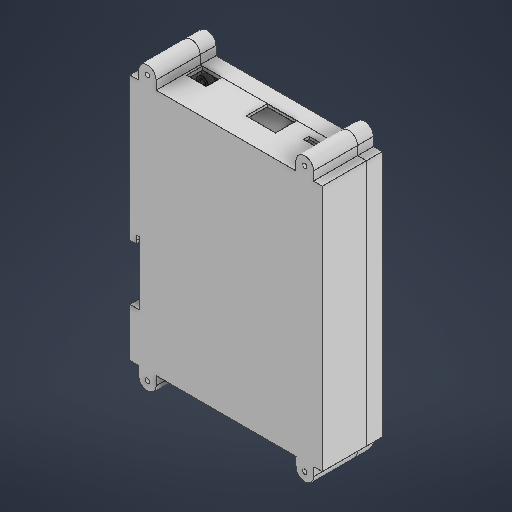
# Autodesk Inventor part: module_base
Saved by Autodesk Inventor 2025 (Build 290162000, 162)
## iProperties
Created: 2024-08-31
Part Number: module_base
Material: Generic
Document SubType Name: Modeling
Designer: Dawid
Density: 1 g/cm^3
Appearance: Default
Author: Dawid
Autodesk Inventor part; units mm, degrees
ref_plane "YZ Plane" through (0, 0, 0) normal (1, 0, 0) x (0, 1, 0)
ref_plane "XZ Plane" through (0, 0, 0) normal (0, 1, 0) x (-1, 0, 0)
ref_plane "XY Plane" through (0, 0, 0) normal (0, 0, 1) x (1, 0, 0)
sketch "Sketch1" plane through (0, 0, 0) normal (0, 0, 1) x (1, 0, 0)
  line L0 (0, 0) -> (70, 0) construction
  line L1 (70, 0) -> (70, 133.34) construction
  line L2 (70, 133.34) -> (0, 133.34) construction
  line L3 (0, 133.34) -> (0, 0) construction
  line L4 (-0.5, 133.84) -> (70.5, 133.84)
  line L5 (70.5, 133.84) -> (70.5, -3)
  line L6 (70.5, -3) -> (-26.344, -3)
  line L7 (-26.344, -3) -> (-26.344, 133.34)
  line L8 (-17.884, 58.58) -> (-12.804, 58.58) construction
  line L9 (-12.804, 58.58) -> (-12.804, 22.58) construction
  line L10 (-12.804, 22.58) -> (-17.884, 22.58) construction
  line L11 (-17.884, 22.58) -> (-17.884, 58.58) construction
  line L12 (-35.844, 135.34) -> (73.5, 135.34)
  line L13 (73.5, 135.34) -> (73.5, -5)
  line L14 (73.5, -5) -> (-35.844, -5)
  line L15 (-31.844, 58.58) -> (-30.344, 58.58)
  line L16 (-30.344, 58.58) -> (-30.344, 22.58)
  line L17 (-30.344, 22.58) -> (-35.844, 22.58)
  line L18 (-35.844, 54.08) -> (-35.844, 135.34)
  line L19 (-35.844, 54.08) -> (-32.144, 54.08)
  line L20 (-31.844, 56.08) -> (-31.844, 58.58)
  line L21 (-35.844, -5) -> (-35.844, 22.58)
  line L22 (-32.144, 54.08) -> (-31.844, 56.08)
  line L23 (-27, 133.34) -> (-1, 133.34) construction
  line L24 (-1, 133.34) -> (-1, 81.44) construction
  line L25 (-1, 81.44) -> (-27, 81.44) construction
  line L26 (-27, 81.44) -> (-27, 133.34) construction
  line L27 (-26.094, 68.63) -> (-4.594, 68.63) construction
  line L28 (-4.594, 68.63) -> (-4.594, 12.53) construction
  line L29 (-4.594, 12.53) -> (-26.094, 12.53) construction
  line L30 (-26.094, 12.53) -> (-26.094, 68.63) construction
  circle A0 centre (-21.62, 124.84) radius 3.5
  circle A1 centre (-6.38, 124.84) radius 3.5
  circle A2 centre (-21.62, 86.74) radius 3.5
  circle A3 centre (-6.38, 86.74) radius 3.5
  circle A4 centre (-21.694, 64.71) radius 3.5
  circle A5 centre (-8.994, 64.71) radius 3.5
  circle A6 centre (-21.694, 16.45) radius 3.5
  circle A7 centre (-8.994, 16.45) radius 3.5
  line L31 (-21.694, 64.71) -> (-8.994, 16.45) construction
  line L32 (-21.62, 124.84) -> (-6.38, 86.74) construction
  circle A8 centre (12.14, 104.13) radius 3.5
  circle A9 centre (57.86, 104.13) radius 3.5
  circle A10 centre (10.87, 29.26) radius 3.5
  circle A11 centre (59.13, 27.96) radius 3.5
  circle A12 centre (26.11, 80.06) radius 3.5
  line L33 (12.14, 104.13) -> (57.86, 104.13) construction
  line L34 (10.87, 29.26) -> (59.13, 29.26) construction
  line L35 (59.13, 29.26) -> (59.13, 27.96) construction
  line L36 (-26.344, 133.34) -> (-0.5, 133.34)
  line L37 (-0.5, 133.34) -> (-0.5, 133.84)
  line L38 (-12.604, 58.78) -> (-18.084, 58.78)
  line L39 (-18.084, 58.78) -> (-18.084, 22.38)
  line L40 (-18.084, 22.38) -> (-12.604, 22.38)
  line L41 (-12.604, 22.38) -> (-12.604, 58.78)
  point P0 (-15.344, 58.58)
  point P1 (-12.804, 40.58)
  point P2 (-15.344, 22.58)
  point P3 (-33.994, 54.08)
  point P4 (-30.344, 40.58)
  point P5 (-15.344, 40.58)
  point P6 (-4.594, 40.58)
  point P7 (-15.344, 12.53)
  point P8 (-14, 105.79)
  point P9 (-14, 81.44)
  point P10 (35, 104.13)
  point P11 (35, 133.34)
  point P12 (35, 29.26)
  dimension "d9" = 70
  dimension "d75" = 0.5
  dimension "d76" = 0.5
  dimension "d77" = 3
  dimension "d83" = 36
  dimension "d84" = 5.08
  dimension "d87" = 3
  dimension "d88" = 1.5
  dimension "d89" = 2
  dimension "d117" = 36
  dimension "d118" = 1.5
  dimension "d121" = 0.3
  dimension "d122" = 2
  dimension "d123" = 4.5
  dimension "d124" = 4
  dimension "d125" = 15
  dimension "d126" = 4
  dimension "d147" = 48.26
  dimension "d148" = 12.7
  dimension "d149" = 56.1
  dimension "d150" = 7
  dimension "d151" = 21.5
  dimension "d152" = 7
  dimension "d153" = 51.9
  dimension "d154" = 26
  dimension "d155" = 15.24
  dimension "d156" = 38.1
  dimension "d158" = 5
  dimension "d159" = 1
  dimension "d160" = 0.5
  dimension "d163" = 7
  dimension "d164" = 45.72
  dimension "d165" = 48.26
  dimension "d166" = 1.3
  dimension "d167" = 24.07
  dimension "d168" = 13.97
  dimension "d169" = 29.21
  dimension "d170" = 76.17
  dimension "d171" = 133.34
  dimension "d182" = 96.844
  dimension "d183" = 45.58
  dimension "d184" = 2
  dimension "d185" = 0.5
  dimension "d215" = 0.2
  constraints: 84 end point, 16 parallel, 13 centre point, 13 midpoint, 11 horizontal, 10 equal radius, 9 perpendicular, 9 vertical alignment, 7 horizontal alignment, 1 collinear, 1 vertical, 3 other
  measures "d9" distance of L1.end L2.end
  measures "d75" distance between parallel lines of L5 L1
  measures "d76" distance between parallel lines of L4 L2
  measures "d77" distance between parallel lines of L6 L0
  measures "d83" distance of L10.end L8.start
  measures "d84" distance of L8.start L8.end
  measures "d87" distance between parallel lines of L13 L5
  measures "d88" distance between parallel lines of L12 L4
  measures "d89" distance between parallel lines of L14 L6
  measures "d117" distance of L15.end L16.end
  measures "d118" distance of L15.start L15.end
  measures "d121" distance from line of L20 L19.end
  measures "d122" vertical distance of L19.end L20.start
  measures "d123" distance from line of point (-33.994, 54.08) L15
  measures "d124" distance between parallel lines of L18 L20
  measures "d125" distance from line of point (-15.344, 58.58) L16
  measures "d126" distance between parallel lines of L7 L16
  measures "d147" distance of L31.end A5.centre
  measures "d148" distance of L31.start A5.centre
  measures "d149" distance of L27.end L28.end
  measures "d150" diameter of A4
  measures "d151" distance of L27.start L27.end
  measures "d152" diameter of A0
  measures "d153" distance of L23.end L24.end
  measures "d154" distance of L24.end L25.end
  measures "d155" distance of L32.end A2.centre
  measures "d156" distance of L32.end A1.centre
  measures "d158" distance edge to line of A1 L23
  measures "d159" distance between parallel lines of L3 L24
  measures "d160" distance between parallel lines of L4 L23
  measures "d163" diameter of A8
  measures "d164" distance of L33.start L33.end
  measures "d165" horizontal distance of L35.end L34.start
  measures "d166" vertical distance of L35.end L34.start
  measures "d167" vertical distance of L33.start A12.centre
  measures "d168" horizontal distance of L33.start A12.centre
  measures "d169" distance from line of L2 L33.end
  measures "d170" vertical distance of L33.end L35.end
  measures "d171" distance of L2.end L0.start
  measures "d182" distance between parallel lines of L5 L7
  measures "d183" distance from line of L14 point (-15.344, 40.58)
  measures "d184" distance between parallel lines of L12 L36
  measures "d185" distance between parallel lines of L37 L3
  measures "d215" distance between parallel lines of L8 L38
extrude "Extrusion1" add sketch "Sketch1" against normal blind 3 contours L4 L5 L6 L7 L36 L37 | L12 L13 L14 L21 L17 L16 L15 L20 L22 L19 L18 | A0 | A1 | A2 | A3 | A4 | A5 | A6 | A7 | A8 | A9 | A10 | A11 | A12 | L41 L40 L39 L38
extrude "Extrusion14" add sketch "Sketch1" along normal blind 4 contours A0 | A1 | A2 | A3 | A4 | A5 | A6 | A7
extrude "Extrusion17" add sketch "Sketch1" along normal blind 9 contours A8 | A9 | A10 | A11 | A12
sketch "Sketch19" plane through (12.14, 104.13, 9) normal (0, 0, 1) x (1, 0, 0)
  circle A0 centre (0, 0) radius 3.5 projected
  circle A1 centre (45.72, 0) radius 3.5 projected
  circle A2 centre (-1.27, -74.87) radius 3.5 projected
  circle A3 centre (46.99, -76.17) radius 3.5 projected
  line L0 (-2.4495, -2.5) -> (2.4495, -2.5)
  line L1 (-3.7195, -72.37) -> (1.1795, -72.37)
  circle A4 centre (46.99, -76.17) radius 3.5 projected
  line L2 (44.5405, -73.67) -> (49.4395, -73.67)
  line L3 (43.2705, -2.5) -> (48.1695, -2.5)
  point P0 (-12.14, -104.13)
  dimension "d186" = 2.5
  dimension "d187" = 2.5
  dimension "d188" = 2.5
  dimension "d189" = 2.5
  constraints: 8 end point, 8 point on circle, 3 horizontal, 1 parallel
  measures "d186" distance from line of A0.centre L0
  measures "d187" distance from line of A2.centre L1
  measures "d188" distance from line of A3.centre L2
  measures "d189" distance from line of L3 A1.centre
extrude "Extrusion18" cut sketch "Sketch19" against normal up to surface (9 mm away) contours L0 A0 | L3 A1 | L1 A2 | L2 A3 picked at (-0.6135, -2.659) picked at (45.1065, -2.659) picked at (-1.8835, -72.211) picked at (46.3765, -73.511)
extrude "Extrusion16" add sketch "Sketch1" along normal blind 6 contours L12 L13 L14 L21 L17 L16 L15 L20 L22 L19 L18
sketch "Sketch10" plane through (0, 0, -3) normal (0, 0, -1) x (-1, 0, 0)
  line L0 (35.844, 135.34) -> (-73.5, 135.34) projected
  line L1 (-73.5, -5) -> (35.844, -5) projected
  line L2 (-68.5, 140.34) -> (-68.5, 135.34)
  line L3 (-58.5, 135.34) -> (-58.5, 140.34)
  arc A0 (-58.5, 140.34) -> (-68.5, 140.34) centre (-63.5, 140.34) ccw
  line L4 (20.844, 140.34) -> (20.844, 135.34)
  line L5 (30.844, 135.34) -> (30.844, 140.34)
  arc A1 (30.844, 140.34) -> (20.844, 140.34) centre (25.844, 140.34) ccw
  line L6 (-68.5, -5) -> (-68.5, -10)
  line L7 (-58.5, -10) -> (-58.5, -5)
  arc A2 (-68.5, -10) -> (-58.5, -10) centre (-63.5, -10) ccw
  line L8 (20.844, -5) -> (20.844, -10)
  line L9 (30.844, -10) -> (30.844, -5)
  arc A3 (20.844, -10) -> (30.844, -10) centre (25.844, -10) ccw
  dimension "d133" = 10
  dimension "d134" = 5
  dimension "d135" = 5
  dimension "d136" = 5
  dimension "d137" = 5
  constraints: 16 end point, 8 point on circle, 8 point on line, 8 tangent, 4 centre point, 4 parallel, 4 vertical, 3 equal radius, 2 horizontal alignment, 2 vertical alignment
  measures "d133" diameter of A0
  measures "d134" distance from line of L0.end L2
  measures "d135" distance from line of L0.start L5
  measures "d136" distance from line of L0 A0.centre
  measures "d137" distance from line of A2.centre L1
extrude "Extrusion9" add sketch "Sketch10" against normal up to surface (9 mm away)
sketch "Sketch17" plane through (7.112, 79.756, 4) normal (0, 0, 1) x (1, 0, 0)
  circle A0 centre (-28.732, 45.084) radius 3.5 projected
  circle A1 centre (-13.492, 45.084) radius 3.5 projected
  circle A2 centre (-28.732, 6.984) radius 3.5 projected
  circle A3 centre (-13.492, 6.984) radius 3.5 projected
  circle A4 centre (-28.806, -15.046) radius 3.5 projected
  circle A5 centre (-16.106, -15.046) radius 3.5 projected
  circle A6 centre (-28.806, -63.306) radius 3.5 projected
  circle A7 centre (-16.106, -63.306) radius 3.5 projected
  point P0 (-28.806, -15.046)
  point P1 (-16.106, -15.046)
  point P2 (-28.806, -63.306)
  point P3 (-16.106, -63.306)
  constraints: 8 coincident
hole "Hole3" at (-8.994, 64.71, 4) at (-21.694, 64.71, 4) at (-6.38, 86.74, 4) at (-21.62, 86.74, 4) at (-21.62, 124.84, 4) at (-8.994, 16.45, 4) at (-21.694, 16.45, 4) at (-6.38, 124.84, 4) direction (0, 0, -1) diameter 3 depth 4 tip angle 118 countersink diameter 4 countersink angle 90
sketch "Sketch18" plane through (12.14, 104.13, 9) normal (0, 0, 1) x (1, 0, 0)
  arc A0 (2.4495, -2.5) -> (-2.4495, -2.5) centre (0, 0) ccw projected
  arc A1 (48.1695, -2.5) -> (43.2705, -2.5) centre (45.72, 0) ccw projected
  arc A2 (-3.7195, -72.37) -> (1.1795, -72.37) centre (-1.27, -74.87) ccw projected
  arc A3 (44.5405, -73.67) -> (49.4395, -73.67) centre (46.99, -76.17) ccw projected
  circle A4 centre (13.97, -24.07) radius 3.5 projected
  line L0 (49.4395, -73.67) -> (44.5405, -73.67) projected
  line L1 (1.1795, -72.37) -> (-3.7195, -72.37) projected
  line L2 (43.2705, -2.5) -> (48.1695, -2.5) projected
  line L3 (-2.4495, -2.5) -> (2.4495, -2.5) projected
  point P0 (-12.14, -104.13)
  constraints: 5 coincident
hole "Hole4" at (59.13, 27.96, 9) at (10.87, 29.26, 9) at (57.86, 104.13, 9) at (12.14, 104.13, 9) at (26.11, 80.06, 9) direction (0, 0, -1) diameter 3 depth 9 tip angle 118 countersink diameter 4 countersink angle 90
sketch "Sketch9" plane through (0, 0, 6) normal (0, 0, 1) x (1, 0, 0)
  circle A0 centre (26.11, 80.06) radius 1.5 projected
  circle A1 centre (12.14, 104.13) radius 1.5 projected
  circle A2 centre (57.86, 104.13) radius 1.5 projected
  circle A3 centre (10.87, 29.26) radius 1.5 projected
  circle A4 centre (59.13, 27.96) radius 1.5 projected
  line L0 (-0.5, 133.84) -> (-0.5, 133.34) projected
  line L1 (-0.5, 133.34) -> (-26.344, 133.34) projected
  line L2 (-26.344, 133.34) -> (-26.344, -3) projected
  line L3 (-26.344, -3) -> (70.5, -3) projected
  line L4 (70.5, -3) -> (70.5, 133.84) projected
  line L5 (70.5, 133.84) -> (-0.5, 133.84) projected
  line L6 (-31.844, 56.08) -> (-32.144, 54.08) projected
  line L7 (-32.144, 54.08) -> (-35.844, 54.08) projected
  line L8 (-35.844, 54.08) -> (-35.844, 135.34) projected
  line L9 (-35.844, 135.34) -> (-30.844, 135.34) projected
  line L10 (-30.844, 135.34) -> (-30.844, 140.34) projected
  arc A5 (-20.844, 140.34) -> (-30.844, 140.34) centre (-25.844, 140.34) ccw projected
  line L11 (-20.844, 140.34) -> (-20.844, 135.34) projected
  line L12 (-20.844, 135.34) -> (58.5, 135.34) projected
  line L13 (58.5, 135.34) -> (58.5, 140.34) projected
  arc A6 (68.5, 140.34) -> (58.5, 140.34) centre (63.5, 140.34) ccw projected
  line L14 (68.5, 140.34) -> (68.5, 135.34) projected
  line L15 (68.5, 135.34) -> (73.5, 135.34) projected
  line L16 (73.5, 135.34) -> (73.5, -5) projected
  line L17 (73.5, -5) -> (68.5, -5) projected
  line L18 (68.5, -5) -> (68.5, -10) projected
  arc A7 (58.5, -10) -> (68.5, -10) centre (63.5, -10) ccw projected
  line L19 (58.5, -10) -> (58.5, -5) projected
  line L20 (58.5, -5) -> (-20.844, -5) projected
  line L21 (-20.844, -5) -> (-20.844, -10) projected
  arc A8 (-30.844, -10) -> (-20.844, -10) centre (-25.844, -10) ccw projected
  line L22 (-30.844, -10) -> (-30.844, -5) projected
  line L23 (-30.844, -5) -> (-35.844, -5) projected
  line L24 (-35.844, -5) -> (-35.844, 22.58) projected
  line L25 (-35.844, 22.58) -> (-30.344, 22.58) projected
  line L26 (-30.344, 22.58) -> (-30.344, 58.58) projected
  line L27 (-30.344, 58.58) -> (-31.844, 58.58) projected
  line L28 (-31.844, 58.58) -> (-31.844, 56.08) projected
  arc A9 (60.3095, 101.63) -> (55.4105, 101.63) centre (57.86, 104.13) ccw projected
  arc A10 (8.4205, 31.76) -> (13.3195, 31.76) centre (10.87, 29.26) ccw projected
  circle A11 centre (26.11, 80.06) radius 3.5 projected
  arc A12 (56.6805, 30.46) -> (61.5795, 30.46) centre (59.13, 27.96) ccw projected
  arc A13 (14.5895, 101.63) -> (9.6905, 101.63) centre (12.14, 104.13) ccw projected
  line L29 (8.4205, 31.76) -> (13.3195, 31.76) projected
  line L30 (14.5895, 101.63) -> (9.6905, 101.63) projected
  line L31 (56.6805, 30.46) -> (61.5795, 30.46) projected
  line L32 (60.3095, 101.63) -> (55.4105, 101.63) projected
extrude "Extrusion7" add sketch "Sketch9" along normal blind 25 separate body contours L6 L7 L8 L9 L10 A5 L11 L12 L13 A6 L14 L15 L16 L17 L18 A7 L19 L20 L21 A8 L22 L23 L24 L25 L26 L27 L28
sketch "Sketch11" plane through (0, 0, 31) normal (0, 0, 1) x (1, 0, 0)
  line L0 (-0.5, 133.84) -> (-0.5, 133.34) projected
  line L1 (-0.5, 133.34) -> (-26.344, 133.34) projected
  line L2 (-26.344, 133.34) -> (-26.344, -3) projected
  line L3 (-26.344, -3) -> (70.5, -3) projected
  line L4 (70.5, -3) -> (70.5, 133.84) projected
  line L5 (70.5, 133.84) -> (-0.5, 133.84) projected
  arc A0 (-30.844, -10) -> (-20.844, -10) centre (-25.844, -10) ccw projected
  line L6 (-30.844, -10) -> (-30.844, -5) projected
  line L7 (-30.844, -5) -> (-35.844, -5) projected
  line L8 (-35.844, -5) -> (-35.844, 22.58) projected
  line L9 (-35.844, 22.58) -> (-30.344, 22.58) projected
  line L10 (-30.344, 22.58) -> (-30.344, 58.58) projected
  line L11 (-30.344, 58.58) -> (-31.844, 58.58) projected
  line L12 (-31.844, 58.58) -> (-31.844, 56.08) projected
  line L13 (-31.844, 56.08) -> (-32.144, 54.08) projected
  line L14 (-32.144, 54.08) -> (-35.844, 54.08) projected
  line L15 (-35.844, 54.08) -> (-35.844, 135.34) projected
  line L16 (-35.844, 135.34) -> (-30.844, 135.34) projected
  line L17 (-30.844, 135.34) -> (-30.844, 140.34) projected
  arc A1 (-20.844, 140.34) -> (-30.844, 140.34) centre (-25.844, 140.34) ccw projected
  line L18 (-20.844, 140.34) -> (-20.844, 135.34) projected
  line L19 (-20.844, 135.34) -> (58.5, 135.34) projected
  line L20 (58.5, 135.34) -> (58.5, 140.34) projected
  arc A2 (68.5, 140.34) -> (58.5, 140.34) centre (63.5, 140.34) ccw projected
  line L21 (68.5, 140.34) -> (68.5, 135.34) projected
  line L22 (68.5, 135.34) -> (73.5, 135.34) projected
  line L23 (73.5, 135.34) -> (73.5, -5) projected
  line L24 (73.5, -5) -> (68.5, -5) projected
  line L25 (68.5, -5) -> (68.5, -10) projected
  arc A3 (58.5, -10) -> (68.5, -10) centre (63.5, -10) ccw projected
  line L26 (58.5, -10) -> (58.5, -5) projected
  line L27 (58.5, -5) -> (-20.844, -5) projected
  line L28 (-20.844, -5) -> (-20.844, -10) projected
extrude "Extrusion10" add sketch "Sketch11" against normal blind 3 contours L5 L4 L3 L2 L1 L0 bodies 2
sketch "Sketch21" plane through (0, 0, -3) normal (0, 0, -1) x (-1, 0, 0)
  arc A0 (-68.5, -10) -> (-58.5, -10) centre (-63.5, -10) ccw projected
  arc A1 (20.844, -10) -> (30.844, -10) centre (25.844, -10) ccw projected
  arc A2 (-58.5, 140.34) -> (-68.5, 140.34) centre (-63.5, 140.34) ccw projected
  arc A3 (30.844, 140.34) -> (20.844, 140.34) centre (25.844, 140.34) ccw projected
  circle A4 centre (-63.5, 140.34) radius 3.5
  circle A5 centre (25.844, 140.34) radius 3.5
  circle A6 centre (-63.5, -10) radius 3.5
  arc A7 (20.844, -10) -> (30.844, -10) centre (25.844, -10) ccw projected
  circle A8 centre (25.844, -10) radius 3.5
  point P0 (0, 0)
  dimension "d212" = 7
  constraints: 4 centre point, 4 coincident, 3 equal radius
  measures "d212" diameter of A4
extrude "Extrusion20" cut sketch "Sketch21" against normal blind 5 bodies 1
sketch "Sketch15" plane through (0, 0, 2) normal (0, 0, -1) x (-1, 0, 0)
  arc A0 (-58.5, 140.34) -> (-68.5, 140.34) centre (-63.5, 140.34) ccw projected
  arc A1 (30.844, 140.34) -> (20.844, 140.34) centre (25.844, 140.34) ccw projected
  arc A2 (20.844, -10) -> (30.844, -10) centre (25.844, -10) ccw projected
  arc A3 (-68.5, -10) -> (-58.5, -10) centre (-63.5, -10) ccw projected
  constraints: 4 coincident
hole "Hole1" at (63.5, -10, 2) at (-25.844, -10, 2) at (-25.844, 140.34, 2) at (63.5, 140.34, 2) direction (0, 0, 1) diameter 3.1 end through all countersink diameter 7 countersink angle 90 bodies 1
sketch "Sketch16" plane through (0, 0, 6) normal (0, 0, -1) x (-1, 0, 0)
  circle A0 centre (-63.5, 140.34) radius 3.5 projected
  circle A1 centre (25.844, 140.34) radius 3.5 projected
  circle A2 centre (-63.5, -10) radius 3.5 projected
  circle A3 centre (25.844, -10) radius 3.5 projected
  constraints: 4 coincident
hole "Hole2" at (-25.844, -10, 6) at (63.5, -10, 6) at (-25.844, 140.34, 6) at (63.5, 140.34, 6) direction (0, 0, 1) diameter 2.6 end through all countersink diameter 3.1 countersink angle 90 bodies 2
extrude "Extrusion15" cut sketch "Sketch1" along normal through all both and the other way through all contours L41 L40 L39 L38 bodies 1
sketch "Sketch20" plane through (-20.844, 135.34, -3) normal (0, 1, 0) x (1, 0, 0)
  line L0 (20.844, -3) -> (90.844, -3) construction
  line L1 (20.844, -9) -> (90.844, -9) construction
  line L2 (90.844, -9) -> (90.844, -10.8) construction
  line L3 (90.844, -10.8) -> (20.844, -10.8) construction
  line L4 (20.844, -10.8) -> (20.844, -9) construction
  line L5 (38.208, -9.2) -> (54.908, -9.2)
  line L6 (54.908, -9.2) -> (54.908, -21.1)
  line L7 (54.908, -21.1) -> (38.208, -21.1)
  line L8 (38.208, -21.1) -> (38.208, -9.2)
  line L9 (66.0445, -13.271) -> (74.2445, -13.271)
  line L10 (74.2445, -13.271) -> (74.2445, -16.371)
  line L11 (74.2445, -16.371) -> (66.0445, -16.371)
  line L12 (66.0445, -16.371) -> (66.0445, -13.271)
  line L13 (1.264, -9) -> (12.424, -9)
  line L14 (12.424, -9) -> (12.424, -18)
  line L15 (12.424, -18) -> (1.264, -18)
  line L16 (1.264, -18) -> (1.264, -9)
  line L17 (19.844, -9) -> (-6.156, -9) construction
  line L18 (-6.156, -9) -> (-6.156, -7.5) construction
  line L19 (-6.156, -7.5) -> (19.844, -7.5) construction
  line L20 (19.844, -7.5) -> (19.844, -9) construction
  point P0 (20.844, -3)
  point P1 (20.844, -3)
  point P2 (90.844, -3)
  point P3 (20.844, -9.9)
  point P4 (46.558, -21.1)
  point P5 (70.1445, -16.371)
  point P6 (6.844, -18)
  point P7 (6.844, -7.5)
  dimension "d192" = 6
  dimension "d193" = 1.8
  dimension "d194" = 1.6
  dimension "d195" = 10.3
  dimension "d196" = 16.7
  dimension "d198" = 25.714
  dimension "d199" = 8.2
  dimension "d200" = 3.1
  dimension "d201" = 20.6995
  dimension "d202" = 2.471
  dimension "d205" = 11.16
  dimension "d206" = 9
  dimension "d208" = 4.5
  dimension "d209" = 1.5
  dimension "d210" = 26
  dimension "d211" = 1
  constraints: 42 end point, 10 parallel, 6 horizontal, 5 midpoint, 5 perpendicular, 3 vertical alignment, 1 collinear
  measures "d192" distance between parallel lines of L0 L1
  measures "d193" distance of L1.end L2.end
  measures "d194" distance between parallel lines of L3 L5
  measures "d195" distance between parallel lines of L7 L3
  measures "d196" distance of L6.end L7.end
  measures "d198" distance from line of L4 point (46.558, -21.1)
  measures "d199" distance of L10.end L11.end
  measures "d200" distance of L11.end L9.start
  measures "d201" distance from line of point (70.144, -16.371) L2
  measures "d202" distance between parallel lines of L3 L9
  measures "d205" distance of L14.end L15.end
  measures "d206" distance of L13.end L14.end
  measures "d208" distance between parallel lines of L19 L0
  measures "d209" distance of L19.end L17.start
  measures "d210" distance of L18.end L19.end
  measures "d211" distance between parallel lines of L4 L20
extrude "Extrusion19" cut sketch "Sketch20" against normal blind 14.5 bodies 1 2
